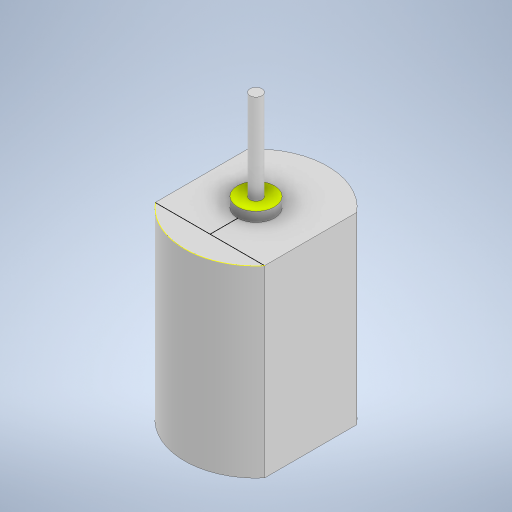
# Autodesk Inventor part: Dc-Motor
Saved by Autodesk Inventor 2024.2 (Build 282272000, 272)
## iProperties
Created: 2023-12-01
Part Number: Dc-Motor
Material: Generic
Document SubType Name: Modeling
Designer: felip
Density: 1 g/cm^3
Appearance: Default
Author: felip
Autodesk Inventor part; units mm, degrees
ref_plane "YZ Plane" through (0, 0, 0) normal (1, 0, 0) x (0, 1, 0)
ref_plane "XZ Plane" through (0, 0, 0) normal (0, 1, 0) x (-1, 0, 0)
ref_plane "XY Plane" through (0, 0, 0) normal (0, 0, 1) x (1, 0, 0)
sketch "Sketch1" plane through (0, 0, 0) normal (0, 1, 0) x (-1, 0, 0)
  point P0 (0, 0)
sketch "Sketch2" plane through (0, 0, 0) normal (0, 1, 0) x (-1, 0, 0)
  arc A0 (9.1, 7.6681) -> (-9.1, 7.6681) centre (0, 0) ccw
  line L0 (0, 0) -> (9.1, 0)
  line L1 (9.1, 0) -> (-9.1, 0)
  line L2 (-9.1, 0) -> (-9.1, -7.6681)
  line L3 (-9.1, 0) -> (-9.1, 7.6681)
  line L4 (9.1, 0) -> (9.1, -7.6681)
  line L5 (9.1, 0) -> (9.1, 7.6681)
  arc A1 (-9.1, -7.6681) -> (9.1, -7.6681) centre (0, 0) ccw
  dimension "d0" = 23.8
  dimension "d1" = 9.1
  dimension "d2" = 18.2
  constraints: 12 end point, 5 point on circle, 3 point on line, 2 centre point, 1 coincident, 1 horizontal, 1 parallel, 1 perpendicular
  measures "d0" diameter of A0
  measures "d1" distance of L0.start L0.end
  measures "d2" distance of L0.end L1.end
extrude "Extrusion1" add sketch "Sketch2" along normal blind 30.6
sketch "Sketch3" plane through (0, 30.6, 0) normal (0, 1, 0) x (1, 0, 0)
  circle A0 centre (0, 0) radius 3.075
  dimension "d5" = 6.15
  constraints: 1 centre point, 1 coincident
  measures "d5" diameter of A0
extrude "Extrusion2" add sketch "Sketch3" along normal blind 1.6
sketch "Sketch4" plane through (0, 32.2, 0) normal (0, 1, 0) x (1, 0, 0)
  circle A0 centre (0, 0) radius 1
  dimension "d8" = 2
  constraints: 1 centre point, 1 coincident
  measures "d8" diameter of A0
extrude "Extrusion3" add sketch "Sketch4" along normal blind 15
sketch "Sketch5" plane through (0, 30.6, 0) normal (0, 1, 0) x (1, 0, 0)
  arc A0 (-9.1, -7.6681) -> (9.1, -7.6681) centre (0, 0) ccw projected
  line L0 (9.1, -7.6681) -> (-9.1, -7.6681)
  circle A1 centre (0, 0) radius 1 projected
  line L1 (0, 0) -> (0, -7.6681)
  constraints: 4 end point, 1 horizontal, 1 midpoint
body "Solid1"
